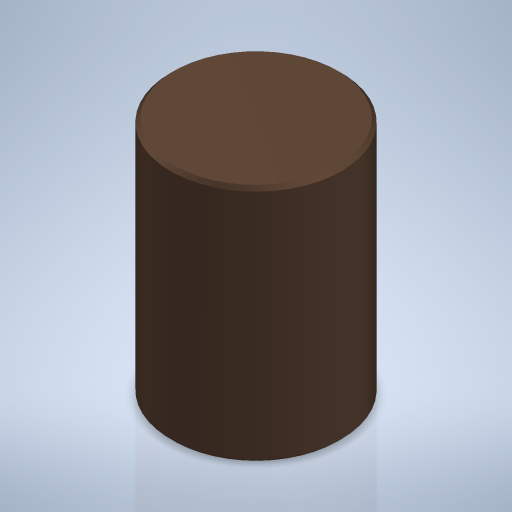
# Autodesk Inventor part: Arbeitskolben
Saved by Autodesk Inventor 2024 (Build 280153000, 153)
## iProperties
Created: 2024-04-02
Part Number: Arbeitskolben
Material: Bronze, Guss
Document SubType Name: Modeling
Designer: ffogue
Density: 8.87 g/cm^3
Appearance: Bronze - satiniert
Author: ffogue
Autodesk Inventor part; units mm, degrees
ref_plane "YZ Plane" through (0, 0, 0) normal (1, 0, 0) x (0, 1, 0)
ref_plane "XZ Plane" through (0, 0, 0) normal (0, 1, 0) x (-1, 0, 0)
sketch "Skizze1" plane through (0, 0, 0) normal (0, 0, 1) x (1, 0, 0)
  circle A0 centre (0, 0) radius 5
  dimension "d0" = 10
  constraints: 1 centre point, 1 coincident
  measures "d0" diameter of A0
extrude "Extrusion1" add sketch "Skizze1" along normal blind 14
sketch "Skizze2" plane through (0, 0, 0) normal (0, 0, -1) x (-1, 0, 0)
  circle A0 centre (0, 0) radius 4
  dimension "d3" = 8
  constraints: 1 centre point, 1 coincident
  measures "d3" diameter of A0
extrude "Extrusion2" cut sketch "Skizze2" against normal blind 7.5
ref_plane "Arbeitsebene1" through (0, 0, 7.5) normal (0, 0, 1) x (1, 0, 0)
sketch "Skizze3" plane through (0, 0, 7.5) normal (0, 0, 1) x (1, 0, 0)
  point P0 (0, 0)
  point P1 (0, 0)
  constraints: 1 coincident
hole "Bohrung1" at (0, 0, 7.5) direction (0, 0, 1) diameter 1.5 depth 4.5 tip angle 118
chamfer "Fasen1" distance 0.2 angle 45 3 edges at (4, 0, 0) (-5, 0, 0) (-5, 0, 14)
